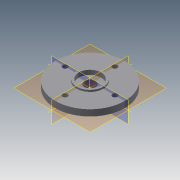
# Autodesk Inventor part: HbServoHorn01
Saved by Autodesk Inventor 2015 SP1 (Build 190203100, 203)
## iProperties
Created: 2015-02-14
Part Number: HbServoHorn01
Material: 一般
Document SubType Name: Modeling
Designer: Yamaura
Density: 1 g/cm^3
Appearance: 既定
Author: Yamaura
Autodesk Inventor part; units mm, degrees
sketch "スケッチ1" plane through (0, 0, 0) normal (0, 0, 1) x (1, 0, 0)
  circle A0 centre (0, 0) radius 10.85
  dimension "d0" = 21.7
  constraints: 1 centre point, 1 coincident
  measures "d0" diameter of A0
extrude "押し出し1" add sketch "スケッチ1" along normal blind 1.95
sketch "スケッチ2" plane through (0, 0, 0) normal (0, 0, 1) x (1, 0, 0)
  circle A0 centre (0, 0) radius 4.7
  dimension "d3" = 9.4
  constraints: 1 centre point, 1 coincident
  measures "d3" diameter of A0
extrude "押し出し2" add sketch "スケッチ2" against normal blind 3.5
sketch "スケッチ3" plane through (0, 0, 0) normal (0, 0, 1) x (1, 0, 0)
  circle A0 centre (0, 0) radius 3
  dimension "d6" = 6
  constraints: 1 centre point, 1 coincident
  measures "d6" diameter of A0
extrude "押し出し3" cut sketch "スケッチ3" against normal blind 3.5
sketch "スケッチ4" plane through (0, 0, 0) normal (0, 0, 1) x (1, 0, 0)
  circle A0 centre (0, 0) radius 4.2
  dimension "d9" = 8.4
  constraints: 1 centre point, 1 coincident
  measures "d9" diameter of A0
extrude "押し出し4" add sketch "スケッチ4" along normal blind 2.5
sketch "スケッチ5" plane through (0, 0, 2.5) normal (0, 0, 1) x (1, 0, 0)
  circle A0 centre (0, 0) radius 3.5
  dimension "d12" = 7
  constraints: 1 centre point, 1 coincident
  measures "d12" diameter of A0
extrude "押し出し5" cut sketch "スケッチ5" against normal blind 1.4
sketch "スケッチ6" plane through (0, 0, 0) normal (0, 0, 1) x (1, 0, 0)
  circle A0 centre (0, 0) radius 1.7
  dimension "d15" = 3.4
  constraints: 1 centre point, 1 coincident
  measures "d15" diameter of A0
extrude "押し出し6" cut sketch "スケッチ6" along normal through all
sketch "スケッチ7" plane through (0, 0, 0) normal (0, 0, 1) x (1, 0, 0)
  circle A0 centre (7.8, 0) radius 0.8
  point P0 (0, 0)
  dimension "d18" = 1.6
  dimension "d19" = 7.8
  constraints: 1 centre point
  measures "d18" diameter of A0
  measures "d19" distance of point (0, 0) A0.centre
extrude "押し出し7" cut sketch "スケッチ7" along normal through all
pattern_circular "円形状パターン1" count 4 over 360 about axis through (0, 0, -10) along (0, 0, 1) of "押し出し7"
chamfer "面取り1" distance 0.2 angle 45 1 edges at (-4.7, 0, 0)
